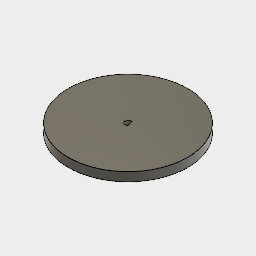
wheel v1 (Autodesk Fusion 360 design; units mm, degrees)
Autodesk Fusion 360 part; units mm, degrees
note: some values were not read from the file. Chosen so that the rebuilt part matches the saved one: which face or edge a step refers to. Set by a fixed rule: which sketch regions a step uses.
sketch "Sketch1" plane through (0, 0, 0) normal (0, 1, 0) x (1, 0, 0) in component "wheel"
  circle A0 centre (43.9449, -41.237) radius 67
  circle A1 centre (43.9449, -41.237) radius 3.5
  dimension "d1" = 134
  dimension "d2" = 7
  measures "d1" diameter of A0
  measures "d2" diameter of A1
extrude "Extrude1" add sketch "Sketch1" along normal blind 10 in component "wheel"
sketch "Sketch2" plane through (0, 10, 0) normal (0, 1, 0) x (-1, 0, 0) in component "wheel"
  circle A0 centre (-43.9449, 41.237) radius 3.5
  circle A1 centre (-43.9449, 41.237) radius 67
  line L0 (-44.9997, 37.8998) -> (-46.3076, 43.8192)
  dimension "d5" = 1.75
  measures "d5" distance of A0.centre L0
extrude "Extrude2" add sketch "Sketch2" against normal blind 10 contours A0 L0 picked at (-46.2468, 41.0806) in component "wheel"
component "wheel" placed x (1, 0, 0) y (0, 1, 0) z (0, 0, 1) at (0, 0, 0)
